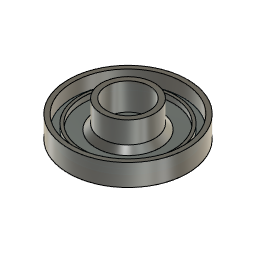
PipeConnector v7 (Autodesk Fusion 360 design; units mm, degrees)
Autodesk Fusion 360 part; units mm, degrees
sketch "Sketch1" plane through (0, 0, 0) normal (0, 0, 1) x (1, 0, 0)
  circle A0 centre (0, 0) radius 10.875
  circle A1 centre (0, 0) radius 12.75
  dimension "d1" = 21.75
  dimension "d2" = 25.5
  constraint coincident A0.centre A1.centre
  constraint concentric A0 A1
  measures "d1" diameter of A0
  measures "d2" diameter of A1
extrude "Extrude1" add sketch "Sketch1" along normal blind 3 makes body 1
sketch "Sketch2" plane through (0, 0, 3) normal (0, 0, 1) x (-1, 0, 0)
  circle A0 centre (0, 0) radius 10.875
  circle A1 centre (0, 0) radius 12.75
  circle A2 centre (0, 0) radius 22
  circle A3 centre (0, 0) radius 5
  constraint coincident A0.centre A1.centre
extrude "Extrude2" add sketch "Sketch2" along normal blind 3 contours A0 | A1 | A2 bodies 1
sketch "Sketch3" plane through (0, 0, 6) normal (0, 0, 1) x (-1, 0, 0)
  circle A0 centre (0, 0) radius 5
  circle A1 centre (0, 0) radius 22
  circle A2 centre (0, 0) radius 7.9
  circle A3 centre (0, 0) radius 9.8005
  circle A4 centre (0, 0) radius 20.3514
  circle A5 centre (0, 0) radius 21.2128
  dimension "d7" = 15.8
  constraint concentric A0 A2
  constraint concentric A0 A3
  constraint concentric A3 A4
  constraint concentric A3 A5
  measures "d7" diameter of A2
extrude "Extrude3" add sketch "Sketch3" along normal blind 5 contours A1 | A3 | A5 bodies 1
extrude "Extrude4" add 1 faces at (-9.1305, 0.4869, 11) along direction (0, 0, 1) blind 5 on bodies 1 bodies 1
sketch "Sketch4" plane through (0, 0, 6) normal (0, 0, 1) x (-1, 0, 0)
  circle A0 centre (0, 0) radius 20.3514
  circle A1 centre (0, 0) radius 9.8005
  circle A2 centre (0, 0) radius 17.7977
  circle A3 centre (0, 0) radius 16.7567
  constraint concentric A0 A2
  constraint coincident A0.centre A1.centre
extrude "Extrude5" add sketch "Sketch4" along normal blind 2 contours A2 bodies 1
sketch "Sketch5" plane through (0, 0, 6) normal (0, 0, 1) x (-1, 0, 0)
  circle A0 centre (0, 0) radius 20.3514
  circle A1 centre (0, 0) radius 17.7977
extrude "Extrude6" add 1 faces at (12.037, -1.1737, 0) along direction (0, 0, -1) blind 3 on bodies 1 bodies 1
chamfer "Chamfer1" distance 3 angle 45 1 edges at (-11.8872, -4.6106, 3) on bodies 1
chamfer "Chamfer2" distance 2 angle 45 1 edges at (9.1373, -3.544, 6) on bodies 1
copy_body "Body->Comp1" bodies 1 removing the originals makes body 2 in component "PipeConnector"
component "PipeConnector" placed x (1, 0, 0) y (0, 1, 0) z (0, 0, 1) at (0, 0, 0)
named bodies: "PipeConnector"
